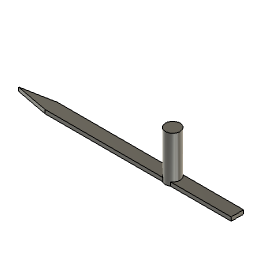
pointer-5 (Autodesk Fusion 360 design; units mm, degrees)
Autodesk Fusion 360 part; units mm, degrees
sketch "草图1" plane through (0, 0, 0) normal (0, 0, 1) x (1, 0, 0)
  line L0 (29.8435, -2) -> (-30.1565, -2)
  line L1 (-30.1565, -2) -> (-30.1565, 2)
  line L2 (-30.1565, 2) -> (29.8435, 2)
  line L3 (29.8435, 2) -> (29.8435, -2)
  line L4 (-30.1565, 2) -> (-40.7091, 0)
  line L5 (-40.7091, 0) -> (-30.1565, -2)
  point P0 (-0.1565, 0)
  dimension "d1" = 60
  dimension "d2" = 4
  constraint horizontal L0
  constraint perpendicular L0 L1
  constraint parallel L0 L2
  constraint parallel L1 L3
  measures "d1" distance of L1.end L2.end
  measures "d2" distance of L0.end L1.end
extrude "拉伸1" add sketch "草图1" along normal blind 1.2
sketch "草图2" plane through (0, 0, 0) normal (0, 0, 1) x (1, 0, 0)
  circle A0 centre (9, 0) radius 2.36
  dimension "d5" = 4.72
  measures "d5" diameter of A0
extrude "拉伸2" add sketch "草图2" along normal blind 14.8
